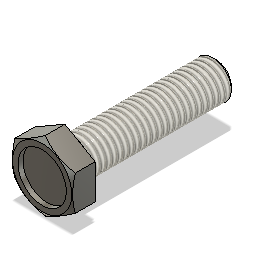
Unmanned Underwater vehicle CAD file (Autodesk Fusion 360 archive; units mm, degrees)
design "Formed Indented Hex Screw ANSI B18.2.3.2M - M10x1.5 x 40 Steel Grade 2 Plain"
description: Formed Indented Hex Screw ANSI B18.2.3.2M - M10x1.5 x 40
part number: FHS ANSI B18.2.3.2M - M10x1.5 x 40 Steel Grade 2 Plain
Autodesk Fusion 360 part; units mm, degrees
sketch "Sketch1" plane through (0, 0, 0) normal (0, 1, 0) x (1, 0, 0)
  line L0 (-5, 39.4) -> (0, 39.4)
  line L1 (0, 39.4) -> (0, -5.304)
  line L2 (-9.24, -0.6) -> (-9.24, -5.8217)
  line L3 (-7.84, -6.63) -> (-6.4, -6.63)
  line L4 (-5, 0) -> (-5, 39.4)
  line L5 (-5, 0) -> (-7.3, 0)
  line L6 (-7.3, 0) -> (-7.3, -0.6)
  line L7 (-7.3, -0.6) -> (-9.24, -0.6)
  line L8 (-6.4, -6.63) -> (-6.4, -5.304)
  line L9 (-6.4, -5.304) -> (0, -5.304)
  line L10 (-9.24, -5.8217) -> (-7.84, -6.63)
  dimension "d81" = 18.48
  dimension "d140" = 14.6
  dimension "d141" = 0.6
  dimension "d151" = 10
  dimension "d156" = 40
  dimension "d160" = 6.63
  dimension "d170" = 30
  dimension "d171" = 15.68
  dimension "d173" = 12.8
  dimension "d175" = 1.326
  constraint vertical L1
  constraint parallel L1 L2
  constraint coincident L1 L9.end
  constraint perpendicular L1 L3
  constraint perpendicular L0 L4
  constraint horizontal L7
  constraint vertical L6
  constraint coincident L4.start L5.start
  constraint coincident origin L5
  constraint coincident L0.start L4.end
  constraint coincident origin L1
  constraint perpendicular L3 L8
  constraint perpendicular L1 L9
  constraint coincident L1.end L9.end
  measures "d141" distance of L5 L7
  measures "d156" distance of L0 L7
  measures "d160" distance of L3 L5
  measures "d170" angle of L3 L10
  measures "d175" distance of L3.end L9
revolve "Revolve1" add sketch "Sketch1" angle 360 about axis through (0, 0, -39.4) along (0, 0, 1)
sketch "Sketch8" plane through (0, 0, 6.63) normal (0, 0, 1) x (1, 0, 0)
  line L0 (-8, -4.6236) -> (-8, 4.6236)
  circle A0 centre (0, 0) radius 9.24
  dimension "d114" = 8
  constraint coincident L0.end A0
  constraint vertical L0
  constraint coincident L0.start A0
  measures "d114" distance of A0.centre L0
extrude "Extrude5" cut sketch "Sketch8" against normal blind 6.63 contours L0 A0 picked at (-8.2001, 1.1262)
pattern_circular "C-Pattern2" count 6 over 360 about axis through (0, 0, 1.75) along (0, 0, 1) of "Extrude5"
thread "Thread3" "ANSI Metric M Profile 10.0 M10x1.5 6g" major diameter 9.85 minor diameter 8.141 pitch 1.5 angle 60 resizes the face on face at (-4.9752, 0.4978, -26.2667) from (0, 0, -1.2404) to (0, 0, -39.4)
sketch "Sketch14" plane through (0, 0, 0) normal (0, 1, 0) x (1, 0, 0)
  line L0 (0, 39.4) -> (0, -5.304)
  line L1 (0, 39.4) -> (-5.1, 39.4)
  line L2 (-5.1, 39.4) -> (-5.1, 38.4)
  line L3 (-5.1, 38.4) -> (-4.1, 39.4)
  dimension "d168" = 45
  dimension "d176" = 4.1
  dimension "d177" = 5.1
  constraint coincident L0.start L1.start
  constraint perpendicular L0 L1
  constraint perpendicular L1 L2
  constraint coincident L1 L3.end
  measures "d168" angle of L2 L3
  measures "d176" distance of L0 L3.end
  measures "d177" distance of L0.start L2
revolve "Revolve4" cut sketch "Sketch14" angle 360 about axis through (0, 0, 1.75) along (0, 0, 1)
equation "adsk_nomlen = 40.00 mm"
equation "adsk_headh = 6.63 mm"
equation "adsk_headdia = 18.48 mm"
equation "adsk_nomdia = 10.00 mm"
equation "d81 = adsk_headdia"
equation "d89 = -adsk_headh"
equation "adsk_waflat = 16.00 mm"
equation "d114 = adsk_waflat / 2"
equation "adsk_thrlen = 38.15965 mm"
equation "adsk_necklen = 0.60 mm"
equation "adsk_beardia = 14.60 mm"
equation "d140 = adsk_beardia"
equation "d141 = adsk_necklen"
equation "adsk_indentdia = adsk_waflat * 0.8"
equation "adsk_indentdepth = adsk_headh * 0.2"
equation "d151 = adsk_nomdia"
equation "d153 = min(adsk_thrlen; adsk_nomlen - adsk_nomdia * 0.1)"
equation "d156 = adsk_nomlen"
equation "d160 = adsk_headh"
equation "d170 = adsk_chamang2"
equation "d171 = adsk_waflat * 0.98"
equation "d173 = adsk_indentdia"
equation "adsk_chamang2 = 30.00 deg"
equation "d175 = adsk_indentdepth"
equation "d176 = d177 - adsk_nomdia * 0.1"
equation "d177 = adsk_nomdia * 0.51"

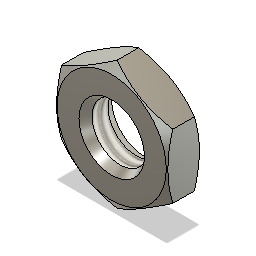
design "Hexagon Thin Nut DIN 439-2 - M10 x 1.5 Steel 6 Plain"
description: Hexagon Thin Nut DIN 439-2 - M10 x 1.5
part number: DIN 439-2 - M10 x 1.5 Steel 6 Plain
Autodesk Fusion 360 part; units mm, degrees
sketch "Sketch1" plane through (0, 0, 0) normal (0, 1, 0) x (1, 0, 0)
  line L0 (0, 0) -> (0, -5)
  line L1 (-5, 0) -> (-8.33, 0)
  line L2 (-8.33, 0) -> (-9.8175, -0.8588)
  line L3 (-9.8175, -0.8588) -> (-9.8175, -4.1412)
  line L4 (-9.8175, -4.1412) -> (-8.33, -5)
  line L5 (-8.33, -5) -> (-5, -5)
  line L6 (-5, -5) -> (-5, 0)
  dimension "d121" = 10
  dimension "d122" = 30
  dimension "d123" = 30
  dimension "d128" = 19.635
  dimension "d172" = 16.66
  dimension "d176" = 5
  constraint vertical L0
  constraint coincident L0 L0.end
  constraint coincident origin L0
  constraint horizontal L1
  constraint perpendicular L1 L3
  constraint perpendicular L3 L5
  constraint perpendicular L5 L6
  constraint coincident L0.start L1
  constraint coincident L0.start origin
  constraint coincident L0.end L5
  constraint vertical L1.end L4.end
  measures "d122" angle of L1 L2
  measures "d123" angle of L4 L5
  measures "d176" distance of L1.start L5
revolve "Revolve1" add sketch "Sketch1" angle 360 about axis through (0, 0, 0) along (0, 0, 1)
sketch "Sketch8" plane through (0, 0, 5) normal (0, 0, 1) x (1, 0, 0)
  line L0 (0, 0) -> (-17, 0) construction
  line L1 (-8.5, -4.9126) -> (-8.5, 4.9126)
  circle A0 centre (0, 0) radius 5
  circle A1 centre (0, 0) radius 9.8175
  dimension "d114" = 8.5
  constraint horizontal L0
  constraint perpendicular L0 L1
  constraint midpoint L0 L1
  constraint coincident L0.start A0.centre
  constraint coincident L1.end A1
  measures "d114" distance of L0.start L1
extrude "Extrude5" cut sketch "Sketch8" against normal blind 5 contours L1 A1 picked at (-8.7126, -1.1966)
pattern_circular "C-Pattern2" count 6 over 360 about axis through (0, 0, 1.75) along (0, 0, 1) of "Extrude5"
thread "Thread3" "ISO Metric profile 10.0 M10x1.5 6H" major diameter 10.198 minor diameter 8.526 pitch 1.5 angle 60 resizes the face on face at (-4.9752, 0.4978, 1.6667)
sketch "Sketch12" plane through (0, 0, 0) normal (0, 1, 0) x (1, 0, 0)
  line L0 (4.263, -5) -> (-4.263, -5)
  line L1 (8.33, -5) -> (-8.33, -5)
  line L2 (8.33, 0) -> (-8.33, 0)
  line L3 (4.263, 0) -> (-4.263, 0)
  line L4 (-5, 0) -> (0, 0)
  line L5 (-3.5566, -2.5) -> (-5, 0)
  line L6 (-5, -5) -> (0, -5)
  line L7 (-3.5566, -2.5) -> (-5, -5)
  line L8 (0, 0) -> (0, -5)
  dimension "d165" = 60
  dimension "d169" = 60
  dimension "d177" = 5
  constraint horizontal L4
  constraint collinear L1 L6
  constraint coincident L5.start L7.start
  constraint vertical L4.start L6.start
  constraint coincident L1 L6.end
  constraint coincident L6.end L8.end
  constraint coincident L4.end L8.start
  measures "d165" angle of L2 L5
  measures "d169" angle of L6 L7
  measures "d177" distance of L4.start L8
revolve "Revolve3" cut sketch "Sketch12" angle 360 about axis through (0, 0, 1.75) along (0, 0, 1)
equation "adsk_nheig = 5.00 mm"
equation "adsk_maxdia = 19.635 mm"
equation "adsk_nomdia = 10.00 mm"
equation "d89 = -adsk_nheig"
equation "adsk_waflat = 17.00 mm"
equation "d114 = adsk_waflat / 2"
equation "adsk_chamang1 = 30.00 deg"
equation "adsk_chamang2 = 30.00 deg"
equation "d121 = adsk_nomdia"
equation "d122 = adsk_chamang1"
equation "d123 = adsk_chamang2"
equation "d128 = adsk_maxdia"
equation "d163 = adsk_nheig"
equation "adsk_beardia = 16.66 mm"
equation "d172 = adsk_beardia"
equation "d176 = adsk_nheig"
equation "d177 = adsk_nomdia * 0.5"

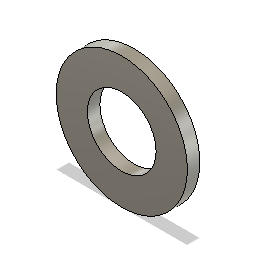
design "Washer BS 4320 - M10 - Form E Steel 100 HV Plain"
description: Washer BS 4320 - M10 - Form E
part number: BW BS 4320 - M10 E Steel 100 HV Plain
Autodesk Fusion 360 part; units mm, degrees
sketch "Sketch1" plane through (0, 0, 0) normal (0, 0, 1) x (1, 0, 0)
  circle A0 centre (0, 0) radius 10.5
  circle A1 centre (0, 0) radius 5.5
  dimension "d4" = 21
  dimension "d5" = 11
  constraint coincident A0.centre A1.centre
  measures "d4" diameter of A0
  measures "d5" diameter of A1
extrude "Extrude1" add sketch "Sketch1" along normal blind 2
equation "adsk_woutdia = 21.00 mm"
equation "adsk_windia = 11.00 mm"
equation "adsk_wthick = 2.00 mm"
equation "d4 = adsk_woutdia"
equation "d5 = adsk_windia"
equation "d6 = adsk_wthick"
equation "d30 = adsk_wthick"

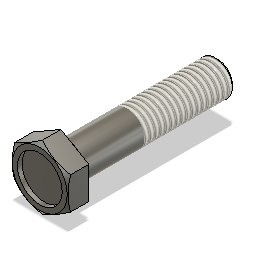
design "Formed Indented Hex Screw ANSI B18.2.3.2M - M10x1.5 x 45 Steel Grade 2 Plain"
description: Formed Indented Hex Screw ANSI B18.2.3.2M - M10x1.5 x 45
part number: FHS ANSI B18.2.3.2M - M10x1.5 x 45 Steel Grade 2 Plain
Autodesk Fusion 360 part; units mm, degrees
sketch "Sketch1" plane through (0, 0, 0) normal (0, 1, 0) x (1, 0, 0)
  line L0 (-5, 44.4) -> (0, 44.4)
  line L1 (0, 44.4) -> (0, -5.304)
  line L2 (-9.24, -0.6) -> (-9.24, -5.8217)
  line L3 (-7.84, -6.63) -> (-6.4, -6.63)
  line L4 (-5, 0) -> (-5, 44.4)
  line L5 (-5, 0) -> (-7.3, 0)
  line L6 (-7.3, 0) -> (-7.3, -0.6)
  line L7 (-7.3, -0.6) -> (-9.24, -0.6)
  line L8 (-6.4, -6.63) -> (-6.4, -5.304)
  line L9 (-6.4, -5.304) -> (0, -5.304)
  line L10 (-9.24, -5.8217) -> (-7.84, -6.63)
  dimension "d81" = 18.48
  dimension "d140" = 14.6
  dimension "d141" = 0.6
  dimension "d151" = 10
  dimension "d156" = 45
  dimension "d160" = 6.63
  dimension "d170" = 30
  dimension "d171" = 15.68
  dimension "d173" = 12.8
  dimension "d175" = 1.326
  constraint vertical L1
  constraint parallel L1 L2
  constraint coincident L1 L9.end
  constraint perpendicular L1 L3
  constraint perpendicular L0 L4
  constraint horizontal L7
  constraint vertical L6
  constraint coincident L4.start L5.start
  constraint coincident origin L5
  constraint coincident L0.start L4.end
  constraint coincident origin L1
  constraint perpendicular L3 L8
  constraint perpendicular L1 L9
  constraint coincident L1.end L9.end
  measures "d141" distance of L5 L7
  measures "d156" distance of L0 L7
  measures "d160" distance of L3 L5
  measures "d170" angle of L3 L10
  measures "d175" distance of L3.end L9
revolve "Revolve1" add sketch "Sketch1" angle 360 about axis through (0, 0, -44.4) along (0, 0, 1)
sketch "Sketch8" plane through (0, 0, 6.63) normal (0, 0, 1) x (1, 0, 0)
  line L0 (-8, -4.6236) -> (-8, 4.6236)
  circle A0 centre (0, 0) radius 9.24
  dimension "d114" = 8
  constraint coincident L0.end A0
  constraint vertical L0
  constraint coincident L0.start A0
  measures "d114" distance of A0.centre L0
extrude "Extrude5" cut sketch "Sketch8" against normal blind 6.63 contours L0 A0 picked at (-8.2001, 1.1262)
pattern_circular "C-Pattern2" count 6 over 360 about axis through (0, 0, 1.75) along (0, 0, 1) of "Extrude5"
thread "Thread3" "ANSI Metric M Profile 10.0 M10x1.5 6g" major diameter 9.85 minor diameter 8.141 pitch 1.5 angle 60 resizes the face on face at (-4.9752, 0.4978, -29.6) from (0, 0, -18.4) to (0, 0, -44.4)
sketch "Sketch14" plane through (0, 0, 0) normal (0, 1, 0) x (1, 0, 0)
  line L0 (0, 44.4) -> (0, -5.304)
  line L1 (0, 44.4) -> (-5.1, 44.4)
  line L2 (-5.1, 44.4) -> (-5.1, 43.4)
  line L3 (-5.1, 43.4) -> (-4.1, 44.4)
  dimension "d168" = 45
  dimension "d176" = 4.1
  dimension "d177" = 5.1
  constraint coincident L0.start L1.start
  constraint perpendicular L0 L1
  constraint perpendicular L1 L2
  constraint coincident L1 L3.end
  measures "d168" angle of L2 L3
  measures "d176" distance of L0 L3.end
  measures "d177" distance of L0.start L2
revolve "Revolve4" cut sketch "Sketch14" angle 360 about axis through (0, 0, 1.75) along (0, 0, 1)
equation "adsk_nomlen = 45.00 mm"
equation "adsk_headh = 6.63 mm"
equation "adsk_headdia = 18.48 mm"
equation "adsk_nomdia = 10.00 mm"
equation "d81 = adsk_headdia"
equation "d89 = -adsk_headh"
equation "adsk_waflat = 16.00 mm"
equation "d114 = adsk_waflat / 2"
equation "adsk_thrlen = 26.00 mm"
equation "adsk_necklen = 0.60 mm"
equation "adsk_beardia = 14.60 mm"
equation "d140 = adsk_beardia"
equation "d141 = adsk_necklen"
equation "adsk_indentdia = adsk_waflat * 0.8"
equation "adsk_indentdepth = adsk_headh * 0.2"
equation "d151 = adsk_nomdia"
equation "d153 = min(adsk_thrlen; adsk_nomlen - adsk_nomdia * 0.1)"
equation "d156 = adsk_nomlen"
equation "d160 = adsk_headh"
equation "d170 = adsk_chamang2"
equation "d171 = adsk_waflat * 0.98"
equation "d173 = adsk_indentdia"
equation "adsk_chamang2 = 30.00 deg"
equation "d175 = adsk_indentdepth"
equation "d176 = d177 - adsk_nomdia * 0.1"
equation "d177 = adsk_nomdia * 0.51"
